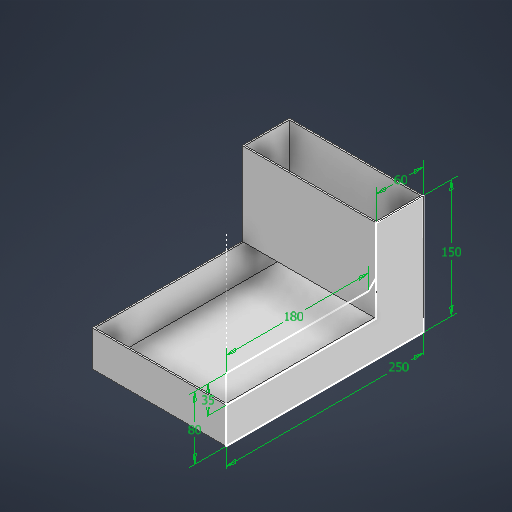
# Autodesk Inventor part: Part1
Saved by Autodesk Inventor 2026.2 (Build 302298000, 298)
## iProperties
Created: 2025-11-07
Part Number: Part1
Material: Generic
Document SubType Name: Modeling
Designer: maxim
Density: 1 g/cm^3
Appearance: Default
Author: maxim
Autodesk Inventor part; units mm, degrees
ref_plane "YZ Plane" through (0, 0, 0) normal (1, 0, 0) x (0, 1, 0)
ref_plane "XZ Plane" through (0, 0, 0) normal (0, 1, 0) x (-1, 0, 0)
ref_plane "XY Plane" through (0, 0, 0) normal (0, 0, 1) x (1, 0, 0)
sketch "Sketch1" plane through (0, 0, 0) normal (1, 0, 0) x (0, 1, 0)
  line L0 (0, 0) -> (80, 0)
  line L1 (80, 0) -> (80, -180)
  line L2 (80, -180) -> (90, -190)
  line L3 (90, -190) -> (150, -190)
  line L4 (150, -190) -> (150, -250)
  line L5 (150, -250) -> (0, -250)
  line L6 (0, -250) -> (0, 0)
  line L7 (45, 0) -> (235, 0) construction
  line L8 (45, -190) -> (45, 0)
  line L9 (90, -190) -> (45, -190)
  dimension "d1" = 150
  dimension "d2" = 60
  dimension "d3" = 180
  dimension "d4" = 80
  dimension "d6" = 250
  dimension "d11" = 35
  constraints: 20 end point, 5 perpendicular, 3 horizontal, 3 point on line, 1 parallel
  measures "d1" distance of L4.end L5.end
  measures "d2" distance of L3.end L4.end
  measures "d3" distance of L0.end L1.end
  measures "d4" distance of L0.start L0.end
  measures "d6" distance of L5.end L0.start
  measures "d11" distance between parallel lines of L8 L1
extrude "Extrusion1" add sketch "Sketch1" against normal blind 170 contours L0 L8 L9 L3 L4 L5 L6
extrude "Extrusion2" add sketch "Sketch1" against normal blind 170 separate body contours L0 L1 L2 L9 L8
shell "Shell1" thickness 2 removed faces 2 at (-113.3333, 86.6667, -186.6667) at (-56.6667, 80, -120)
shell "Shell2" thickness 2 removed faces 3 at (-56.6667, 150, -230) at (-56.6667, 45, -126.6667) at (-56.6667, 45, -63.3333)
body "Solid1"
body "Solid2"
